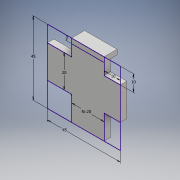
# Autodesk Inventor part: 071_0100_Base
Saved by Autodesk Inventor 2018 (Build 220112000, 112)
## iProperties
Created: 2018-07-06
Part Number: 071_0100_Base
Material: Generic
Document SubType Name: Modeling
Designer: deniz
Density: 1 g/cm^3
Appearance: Default
Author: deniz
Autodesk Inventor part; units mm, degrees
ref_plane "YZ Plane" through (0, 0, 0) normal (1, 0, 0) x (0, 1, 0)
ref_plane "XZ Plane" through (0, 0, 0) normal (0, 1, 0) x (-1, 0, 0)
ref_plane "XY Plane" through (0, 0, 0) normal (0, 0, 1) x (1, 0, 0)
sketch "Sketch1" plane through (0, 0, 0) normal (0, 1, 0) x (-1, 0, 0)
  line L0 (0, 0) -> (45, 0)
  line L1 (45, 0) -> (45, -45)
  line L2 (45, -45) -> (0, -45)
  line L3 (0, -45) -> (0, 0)
  line L4 (30, 0) -> (30, -10)
  line L5 (30, -10) -> (45, -10)
  line L6 (30, -30) -> (30, -45)
  line L7 (30, -30) -> (45, -30)
  line L8 (10, -30) -> (0, -30)
  line L9 (10, -30) -> (10, -45)
  line L10 (10, -10) -> (10, 0)
  line L11 (10, -10) -> (0, -10)
  line L12 (30, -3) -> (10, -3)
  dimension "d2" = 20
  dimension "d8" = 20
  dimension "d9" = 45
  dimension "d10" = 10
  dimension "d11" = 45
  dimension "d12" = 10
  dimension "d13" = 3
  constraints: 26 end point, 17 point on line, 5 perpendicular, 2 parallel, 1 collinear, 1 horizontal, 1 vertical
  measures "d2" distance between parallel lines of L7 L5
  measures "d8" distance between parallel lines of L9 L6
  measures "d9" distance of L1.end L2.end
  measures "d10" distance of L10.start L11.end
  measures "d11" distance between parallel lines of L0 L2
  measures "d12" distance between parallel lines of L0 L11
  measures "d13" distance between parallel lines of L0 L12
extrude "Extrusion1" add sketch "Sketch1" along normal blind 4 contours L0 L4 L12 L10 | L11 L10 L12 L4 L5 L1 L7 L6 L2 L9 L8 L3
fillet "Fillet1" radius 1.8 1 edges at (-30, 2, -30)
extrude "Extrusion3" add sketch "Sketch1" along normal blind 8 contours L0 L4 L12 L10
equation "\"d8\" = d2"
body "Solid1"
